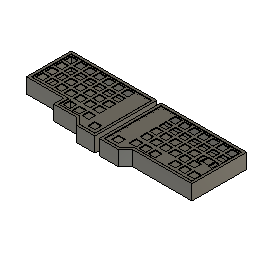
hwsplit (Autodesk Fusion 360 design; units mm, degrees)
Autodesk Fusion 360 part; units mm, degrees
sketch "Sketch1" plane through (0, 0, 0) normal (0, 0, 1) x (1, 0, 0)
  line L0 (3.025, -2.525) -> (16.025, -2.525)
  line L1 (3.025, -16.525) -> (16.025, -16.525)
  line L2 (2.525, -3.025) -> (2.525, -16.025)
  line L3 (16.525, -3.025) -> (16.525, -16.025)
  arc A0 (3.025, -2.525) -> (2.525, -3.025) centre (3.025, -3.025) ccw
  arc A1 (16.525, -3.025) -> (16.025, -2.525) centre (16.025, -3.025) ccw
  arc A2 (2.525, -16.025) -> (3.025, -16.525) centre (3.025, -16.025) ccw
  arc A3 (16.025, -16.525) -> (16.525, -16.025) centre (16.025, -16.025) ccw
  line L4 (22.075, -2.525) -> (35.075, -2.525)
  line L5 (22.075, -16.525) -> (35.075, -16.525)
  line L6 (21.575, -3.025) -> (21.575, -16.025)
  line L7 (35.575, -3.025) -> (35.575, -16.025)
  arc A4 (22.075, -2.525) -> (21.575, -3.025) centre (22.075, -3.025) ccw
  arc A5 (35.575, -3.025) -> (35.075, -2.525) centre (35.075, -3.025) ccw
  arc A6 (21.575, -16.025) -> (22.075, -16.525) centre (22.075, -16.025) ccw
  arc A7 (35.075, -16.525) -> (35.575, -16.025) centre (35.075, -16.025) ccw
  line L8 (41.125, -2.525) -> (54.125, -2.525)
  line L9 (41.125, -16.525) -> (54.125, -16.525)
  line L10 (40.625, -3.025) -> (40.625, -16.025)
  line L11 (54.625, -3.025) -> (54.625, -16.025)
  arc A8 (41.125, -2.525) -> (40.625, -3.025) centre (41.125, -3.025) ccw
  arc A9 (54.625, -3.025) -> (54.125, -2.525) centre (54.125, -3.025) ccw
  arc A10 (40.625, -16.025) -> (41.125, -16.525) centre (41.125, -16.025) ccw
  arc A11 (54.125, -16.525) -> (54.625, -16.025) centre (54.125, -16.025) ccw
  line L12 (60.175, -2.525) -> (73.175, -2.525)
  line L13 (60.175, -16.525) -> (73.175, -16.525)
  line L14 (59.675, -3.025) -> (59.675, -16.025)
  line L15 (73.675, -3.025) -> (73.675, -16.025)
  arc A12 (60.175, -2.525) -> (59.675, -3.025) centre (60.175, -3.025) ccw
  arc A13 (73.675, -3.025) -> (73.175, -2.525) centre (73.175, -3.025) ccw
  arc A14 (59.675, -16.025) -> (60.175, -16.525) centre (60.175, -16.025) ccw
  arc A15 (73.175, -16.525) -> (73.675, -16.025) centre (73.175, -16.025) ccw
  line L16 (79.225, -2.525) -> (92.225, -2.525)
  line L17 (79.225, -16.525) -> (92.225, -16.525)
  line L18 (78.725, -3.025) -> (78.725, -16.025)
  line L19 (92.725, -3.025) -> (92.725, -16.025)
  arc A16 (79.225, -2.525) -> (78.725, -3.025) centre (79.225, -3.025) ccw
  arc A17 (92.725, -3.025) -> (92.225, -2.525) centre (92.225, -3.025) ccw
  arc A18 (78.725, -16.025) -> (79.225, -16.525) centre (79.225, -16.025) ccw
  arc A19 (92.225, -16.525) -> (92.725, -16.025) centre (92.225, -16.025) ccw
  line L20 (98.275, -2.525) -> (111.275, -2.525)
  line L21 (98.275, -16.525) -> (111.275, -16.525)
  line L22 (97.775, -3.025) -> (97.775, -16.025)
  line L23 (111.775, -3.025) -> (111.775, -16.025)
  arc A20 (98.275, -2.525) -> (97.775, -3.025) centre (98.275, -3.025) ccw
  arc A21 (111.775, -3.025) -> (111.275, -2.525) centre (111.275, -3.025) ccw
  arc A22 (97.775, -16.025) -> (98.275, -16.525) centre (98.275, -16.025) ccw
  arc A23 (111.275, -16.525) -> (111.775, -16.025) centre (111.275, -16.025) ccw
  line L24 (117.325, -2.525) -> (130.325, -2.525)
  line L25 (117.325, -16.525) -> (130.325, -16.525)
  line L26 (116.825, -3.025) -> (116.825, -16.025)
  line L27 (130.825, -3.025) -> (130.825, -16.025)
  arc A24 (117.325, -2.525) -> (116.825, -3.025) centre (117.325, -3.025) ccw
  arc A25 (130.825, -3.025) -> (130.325, -2.525) centre (130.325, -3.025) ccw
  arc A26 (116.825, -16.025) -> (117.325, -16.525) centre (117.325, -16.025) ccw
  arc A27 (130.325, -16.525) -> (130.825, -16.025) centre (130.325, -16.025) ccw
  line L28 (212.575, -2.525) -> (225.575, -2.525)
  line L29 (212.575, -16.525) -> (225.575, -16.525)
  line L30 (212.075, -3.025) -> (212.075, -16.025)
  line L31 (226.075, -3.025) -> (226.075, -16.025)
  arc A28 (212.575, -2.525) -> (212.075, -3.025) centre (212.575, -3.025) ccw
  arc A29 (226.075, -3.025) -> (225.575, -2.525) centre (225.575, -3.025) ccw
  arc A30 (212.075, -16.025) -> (212.575, -16.525) centre (212.575, -16.025) ccw
  arc A31 (225.575, -16.525) -> (226.075, -16.025) centre (225.575, -16.025) ccw
  line L32 (231.625, -2.525) -> (244.625, -2.525)
  line L33 (231.625, -16.525) -> (244.625, -16.525)
  line L34 (231.125, -3.025) -> (231.125, -16.025)
  line L35 (245.125, -3.025) -> (245.125, -16.025)
  arc A32 (231.625, -2.525) -> (231.125, -3.025) centre (231.625, -3.025) ccw
  arc A33 (245.125, -3.025) -> (244.625, -2.525) centre (244.625, -3.025) ccw
  arc A34 (231.125, -16.025) -> (231.625, -16.525) centre (231.625, -16.025) ccw
  arc A35 (244.625, -16.525) -> (245.125, -16.025) centre (244.625, -16.025) ccw
  line L36 (250.675, -2.525) -> (263.675, -2.525)
  line L37 (250.675, -16.525) -> (263.675, -16.525)
  line L38 (250.175, -3.025) -> (250.175, -16.025)
  line L39 (264.175, -3.025) -> (264.175, -16.025)
  arc A36 (250.675, -2.525) -> (250.175, -3.025) centre (250.675, -3.025) ccw
  arc A37 (264.175, -3.025) -> (263.675, -2.525) centre (263.675, -3.025) ccw
  arc A38 (250.175, -16.025) -> (250.675, -16.525) centre (250.675, -16.025) ccw
  arc A39 (263.675, -16.525) -> (264.175, -16.025) centre (263.675, -16.025) ccw
  line L40 (269.725, -2.525) -> (282.725, -2.525)
  line L41 (269.725, -16.525) -> (282.725, -16.525)
  line L42 (269.225, -3.025) -> (269.225, -16.025)
  line L43 (283.225, -3.025) -> (283.225, -16.025)
  arc A40 (269.725, -2.525) -> (269.225, -3.025) centre (269.725, -3.025) ccw
  arc A41 (283.225, -3.025) -> (282.725, -2.525) centre (282.725, -3.025) ccw
  arc A42 (269.225, -16.025) -> (269.725, -16.525) centre (269.725, -16.025) ccw
  arc A43 (282.725, -16.525) -> (283.225, -16.025) centre (282.725, -16.025) ccw
  line L44 (288.775, -2.525) -> (301.775, -2.525)
  line L45 (288.775, -16.525) -> (301.775, -16.525)
  line L46 (288.275, -3.025) -> (288.275, -16.025)
  line L47 (302.275, -3.025) -> (302.275, -16.025)
  arc A44 (288.775, -2.525) -> (288.275, -3.025) centre (288.775, -3.025) ccw
  arc A45 (302.275, -3.025) -> (301.775, -2.525) centre (301.775, -3.025) ccw
  arc A46 (288.275, -16.025) -> (288.775, -16.525) centre (288.775, -16.025) ccw
  arc A47 (301.775, -16.525) -> (302.275, -16.025) centre (301.775, -16.025) ccw
  line L48 (307.825, -2.525) -> (320.825, -2.525)
  line L49 (307.825, -16.525) -> (320.825, -16.525)
  line L50 (307.325, -3.025) -> (307.325, -16.025)
  line L51 (321.325, -3.025) -> (321.325, -16.025)
  arc A48 (307.825, -2.525) -> (307.325, -3.025) centre (307.825, -3.025) ccw
  arc A49 (321.325, -3.025) -> (320.825, -2.525) centre (320.825, -3.025) ccw
  arc A50 (307.325, -16.025) -> (307.825, -16.525) centre (307.825, -16.025) ccw
  arc A51 (320.825, -16.525) -> (321.325, -16.025) centre (320.825, -16.025) ccw
  line L52 (326.875, -2.525) -> (339.875, -2.525)
  line L53 (326.875, -16.525) -> (339.875, -16.525)
  line L54 (326.375, -3.025) -> (326.375, -16.025)
  line L55 (340.375, -3.025) -> (340.375, -16.025)
  arc A52 (326.875, -2.525) -> (326.375, -3.025) centre (326.875, -3.025) ccw
  arc A53 (340.375, -3.025) -> (339.875, -2.525) centre (339.875, -3.025) ccw
  arc A54 (326.375, -16.025) -> (326.875, -16.525) centre (326.875, -16.025) ccw
  arc A55 (339.875, -16.525) -> (340.375, -16.025) centre (339.875, -16.025) ccw
  line L56 (3.025, -21.575) -> (16.025, -21.575)
  line L57 (3.025, -35.575) -> (16.025, -35.575)
  line L58 (2.525, -22.075) -> (2.525, -35.075)
  line L59 (16.525, -22.075) -> (16.525, -35.075)
  arc A56 (3.025, -21.575) -> (2.525, -22.075) centre (3.025, -22.075) ccw
  arc A57 (16.525, -22.075) -> (16.025, -21.575) centre (16.025, -22.075) ccw
  arc A58 (2.525, -35.075) -> (3.025, -35.575) centre (3.025, -35.075) ccw
  arc A59 (16.025, -35.575) -> (16.525, -35.075) centre (16.025, -35.075) ccw
  line L60 (22.075, -21.575) -> (35.075, -21.575)
  line L61 (22.075, -35.575) -> (35.075, -35.575)
  line L62 (21.575, -22.075) -> (21.575, -35.075)
  line L63 (35.575, -22.075) -> (35.575, -35.075)
  arc A60 (22.075, -21.575) -> (21.575, -22.075) centre (22.075, -22.075) ccw
  arc A61 (35.575, -22.075) -> (35.075, -21.575) centre (35.075, -22.075) ccw
  arc A62 (21.575, -35.075) -> (22.075, -35.575) centre (22.075, -35.075) ccw
  arc A63 (35.075, -35.575) -> (35.575, -35.075) centre (35.075, -35.075) ccw
  line L64 (41.125, -21.575) -> (54.125, -21.575)
  line L65 (41.125, -35.575) -> (54.125, -35.575)
  line L66 (40.625, -22.075) -> (40.625, -35.075)
  line L67 (54.625, -22.075) -> (54.625, -35.075)
  arc A64 (41.125, -21.575) -> (40.625, -22.075) centre (41.125, -22.075) ccw
  arc A65 (54.625, -22.075) -> (54.125, -21.575) centre (54.125, -22.075) ccw
  arc A66 (40.625, -35.075) -> (41.125, -35.575) centre (41.125, -35.075) ccw
  arc A67 (54.125, -35.575) -> (54.625, -35.075) centre (54.125, -35.075) ccw
  line L68 (60.175, -21.575) -> (73.175, -21.575)
  line L69 (60.175, -35.575) -> (73.175, -35.575)
  line L70 (59.675, -22.075) -> (59.675, -35.075)
  line L71 (73.675, -22.075) -> (73.675, -35.075)
  arc A68 (60.175, -21.575) -> (59.675, -22.075) centre (60.175, -22.075) ccw
  arc A69 (73.675, -22.075) -> (73.175, -21.575) centre (73.175, -22.075) ccw
  arc A70 (59.675, -35.075) -> (60.175, -35.575) centre (60.175, -35.075) ccw
  arc A71 (73.175, -35.575) -> (73.675, -35.075) centre (73.175, -35.075) ccw
  line L72 (79.225, -21.575) -> (92.225, -21.575)
  line L73 (79.225, -35.575) -> (92.225, -35.575)
  line L74 (78.725, -22.075) -> (78.725, -35.075)
  line L75 (92.725, -22.075) -> (92.725, -35.075)
  arc A72 (79.225, -21.575) -> (78.725, -22.075) centre (79.225, -22.075) ccw
  arc A73 (92.725, -22.075) -> (92.225, -21.575) centre (92.225, -22.075) ccw
  arc A74 (78.725, -35.075) -> (79.225, -35.575) centre (79.225, -35.075) ccw
  arc A75 (92.225, -35.575) -> (92.725, -35.075) centre (92.225, -35.075) ccw
  line L76 (98.275, -21.575) -> (111.275, -21.575)
  line L77 (98.275, -35.575) -> (111.275, -35.575)
  line L78 (97.775, -22.075) -> (97.775, -35.075)
  line L79 (111.775, -22.075) -> (111.775, -35.075)
  arc A76 (98.275, -21.575) -> (97.775, -22.075) centre (98.275, -22.075) ccw
  arc A77 (111.775, -22.075) -> (111.275, -21.575) centre (111.275, -22.075) ccw
  arc A78 (97.775, -35.075) -> (98.275, -35.575) centre (98.275, -35.075) ccw
  arc A79 (111.275, -35.575) -> (111.775, -35.075) centre (111.275, -35.075) ccw
  line L80 (117.325, -21.575) -> (130.325, -21.575)
  line L81 (117.325, -35.575) -> (130.325, -35.575)
  line L82 (116.825, -22.075) -> (116.825, -35.075)
  line L83 (130.825, -22.075) -> (130.825, -35.075)
  arc A80 (117.325, -21.575) -> (116.825, -22.075) centre (117.325, -22.075) ccw
  arc A81 (130.825, -22.075) -> (130.325, -21.575) centre (130.325, -22.075) ccw
  arc A82 (116.825, -35.075) -> (117.325, -35.575) centre (117.325, -35.075) ccw
  arc A83 (130.325, -35.575) -> (130.825, -35.075) centre (130.325, -35.075) ccw
  line L84 (212.575, -21.575) -> (225.575, -21.575)
  line L85 (212.575, -35.575) -> (225.575, -35.575)
  line L86 (212.075, -22.075) -> (212.075, -35.075)
  line L87 (226.075, -22.075) -> (226.075, -35.075)
  arc A84 (212.575, -21.575) -> (212.075, -22.075) centre (212.575, -22.075) ccw
  arc A85 (226.075, -22.075) -> (225.575, -21.575) centre (225.575, -22.075) ccw
  arc A86 (212.075, -35.075) -> (212.575, -35.575) centre (212.575, -35.075) ccw
  arc A87 (225.575, -35.575) -> (226.075, -35.075) centre (225.575, -35.075) ccw
  line L88 (231.625, -21.575) -> (244.625, -21.575)
  line L89 (231.625, -35.575) -> (244.625, -35.575)
  line L90 (231.125, -22.075) -> (231.125, -35.075)
  line L91 (245.125, -22.075) -> (245.125, -35.075)
  arc A88 (231.625, -21.575) -> (231.125, -22.075) centre (231.625, -22.075) ccw
  arc A89 (245.125, -22.075) -> (244.625, -21.575) centre (244.625, -22.075) ccw
  arc A90 (231.125, -35.075) -> (231.625, -35.575) centre (231.625, -35.075) ccw
  arc A91 (244.625, -35.575) -> (245.125, -35.075) centre (244.625, -35.075) ccw
  line L92 (250.675, -21.575) -> (263.675, -21.575)
  line L93 (250.675, -35.575) -> (263.675, -35.575)
  line L94 (250.175, -22.075) -> (250.175, -35.075)
  line L95 (264.175, -22.075) -> (264.175, -35.075)
  arc A92 (250.675, -21.575) -> (250.175, -22.075) centre (250.675, -22.075) ccw
  arc A93 (264.175, -22.075) -> (263.675, -21.575) centre (263.675, -22.075) ccw
  arc A94 (250.175, -35.075) -> (250.675, -35.575) centre (250.675, -35.075) ccw
  arc A95 (263.675, -35.575) -> (264.175, -35.075) centre (263.675, -35.075) ccw
  line L96 (269.725, -21.575) -> (282.725, -21.575)
  line L97 (269.725, -35.575) -> (282.725, -35.575)
  line L98 (269.225, -22.075) -> (269.225, -35.075)
  line L99 (283.225, -22.075) -> (283.225, -35.075)
  arc A96 (269.725, -21.575) -> (269.225, -22.075) centre (269.725, -22.075) ccw
  arc A97 (283.225, -22.075) -> (282.725, -21.575) centre (282.725, -22.075) ccw
  arc A98 (269.225, -35.075) -> (269.725, -35.575) centre (269.725, -35.075) ccw
  arc A99 (282.725, -35.575) -> (283.225, -35.075) centre (282.725, -35.075) ccw
  line L100 (288.775, -21.575) -> (301.775, -21.575)
  line L101 (288.775, -35.575) -> (301.775, -35.575)
  line L102 (288.275, -22.075) -> (288.275, -35.075)
  line L103 (302.275, -22.075) -> (302.275, -35.075)
  arc A100 (288.775, -21.575) -> (288.275, -22.075) centre (288.775, -22.075) ccw
  arc A101 (302.275, -22.075) -> (301.775, -21.575) centre (301.775, -22.075) ccw
  arc A102 (288.275, -35.075) -> (288.775, -35.575) centre (288.775, -35.075) ccw
  arc A103 (301.775, -35.575) -> (302.275, -35.075) centre (301.775, -35.075) ccw
  line L104 (307.825, -21.575) -> (320.825, -21.575)
  line L105 (307.825, -35.575) -> (320.825, -35.575)
  line L106 (307.325, -22.075) -> (307.325, -35.075)
  line L107 (321.325, -22.075) -> (321.325, -35.075)
  arc A104 (307.825, -21.575) -> (307.325, -22.075) centre (307.825, -22.075) ccw
  arc A105 (321.325, -22.075) -> (320.825, -21.575) centre (320.825, -22.075) ccw
  arc A106 (307.325, -35.075) -> (307.825, -35.575) centre (307.825, -35.075) ccw
  arc A107 (320.825, -35.575) -> (321.325, -35.075) centre (320.825, -35.075) ccw
  line L108 (326.875, -21.575) -> (339.875, -21.575)
  line L109 (326.875, -35.575) -> (339.875, -35.575)
  line L110 (326.375, -22.075) -> (326.375, -35.075)
  line L111 (340.375, -22.075) -> (340.375, -35.075)
  arc A108 (326.875, -21.575) -> (326.375, -22.075) centre (326.875, -22.075) ccw
  arc A109 (340.375, -22.075) -> (339.875, -21.575) centre (339.875, -22.075) ccw
  arc A110 (326.375, -35.075) -> (326.875, -35.575) centre (326.875, -35.075) ccw
  arc A111 (339.875, -35.575) -> (340.375, -35.075) centre (339.875, -35.075) ccw
  line L112 (3.025, -40.625) -> (16.025, -40.625)
  line L113 (3.025, -54.625) -> (16.025, -54.625)
  line L114 (2.525, -41.125) -> (2.525, -54.125)
  line L115 (16.525, -41.125) -> (16.525, -54.125)
  arc A112 (3.025, -40.625) -> (2.525, -41.125) centre (3.025, -41.125) ccw
  arc A113 (16.525, -41.125) -> (16.025, -40.625) centre (16.025, -41.125) ccw
  arc A114 (2.525, -54.125) -> (3.025, -54.625) centre (3.025, -54.125) ccw
  arc A115 (16.025, -54.625) -> (16.525, -54.125) centre (16.025, -54.125) ccw
  line L116 (22.075, -40.625) -> (35.075, -40.625)
  line L117 (22.075, -54.625) -> (35.075, -54.625)
  line L118 (21.575, -41.125) -> (21.575, -54.125)
  line L119 (35.575, -41.125) -> (35.575, -54.125)
  arc A116 (22.075, -40.625) -> (21.575, -41.125) centre (22.075, -41.125) ccw
  arc A117 (35.575, -41.125) -> (35.075, -40.625) centre (35.075, -41.125) ccw
  arc A118 (21.575, -54.125) -> (22.075, -54.625) centre (22.075, -54.125) ccw
  arc A119 (35.075, -54.625) -> (35.575, -54.125) centre (35.075, -54.125) ccw
  line L120 (41.125, -40.625) -> (54.125, -40.625)
  line L121 (41.125, -54.625) -> (54.125, -54.625)
  line L122 (40.625, -41.125) -> (40.625, -54.125)
  line L123 (54.625, -41.125) -> (54.625, -54.125)
  arc A120 (41.125, -40.625) -> (40.625, -41.125) centre (41.125, -41.125) ccw
  arc A121 (54.625, -41.125) -> (54.125, -40.625) centre (54.125, -41.125) ccw
  arc A122 (40.625, -54.125) -> (41.125, -54.625) centre (41.125, -54.125) ccw
  arc A123 (54.125, -54.625) -> (54.625, -54.125) centre (54.125, -54.125) ccw
  line L124 (60.175, -40.625) -> (73.175, -40.625)
  line L125 (60.175, -54.625) -> (73.175, -54.625)
  line L126 (59.675, -41.125) -> (59.675, -54.125)
  line L127 (73.675, -41.125) -> (73.675, -54.125)
  arc A124 (60.175, -40.625) -> (59.675, -41.125) centre (60.175, -41.125) ccw
  arc A125 (73.675, -41.125) -> (73.175, -40.625) centre (73.175, -41.125) ccw
  arc A126 (59.675, -54.125) -> (60.175, -54.625) centre (60.175, -54.125) ccw
  arc A127 (73.175, -54.625) -> (73.675, -54.125) centre (73.175, -54.125) ccw
  line L128 (79.225, -40.625) -> (92.225, -40.625)
  line L129 (79.225, -54.625) -> (92.225, -54.625)
  line L130 (78.725, -41.125) -> (78.725, -54.125)
  line L131 (92.725, -41.125) -> (92.725, -54.125)
  arc A128 (79.225, -40.625) -> (78.725, -41.125) centre (79.225, -41.125) ccw
  arc A129 (92.725, -41.125) -> (92.225, -40.625) centre (92.225, -41.125) ccw
  arc A130 (78.725, -54.125) -> (79.225, -54.625) centre (79.225, -54.125) ccw
  arc A131 (92.225, -54.625) -> (92.725, -54.125) centre (92.225, -54.125) ccw
  line L132 (98.275, -40.625) -> (111.275, -40.625)
  line L133 (98.275, -54.625) -> (111.275, -54.625)
  line L134 (97.775, -41.125) -> (97.775, -54.125)
  line L135 (111.775, -41.125) -> (111.775, -54.125)
  arc A132 (98.275, -40.625) -> (97.775, -41.125) centre (98.275, -41.125) ccw
  arc A133 (111.775, -41.125) -> (111.275, -40.625) centre (111.275, -41.125) ccw
  arc A134 (97.775, -54.125) -> (98.275, -54.625) centre (98.275, -54.125) ccw
  arc A135 (111.275, -54.625) -> (111.775, -54.125) centre (111.275, -54.125) ccw
  line L136 (117.325, -40.625) -> (130.325, -40.625)
  line L137 (117.325, -54.625) -> (130.325, -54.625)
  line L138 (116.825, -41.125) -> (116.825, -54.125)
  line L139 (130.825, -41.125) -> (130.825, -54.125)
  arc A136 (117.325, -40.625) -> (116.825, -41.125) centre (117.325, -41.125) ccw
  arc A137 (130.825, -41.125) -> (130.325, -40.625) centre (130.325, -41.125) ccw
  arc A138 (116.825, -54.125) -> (117.325, -54.625) centre (117.325, -54.125) ccw
  arc A139 (130.325, -54.625) -> (130.825, -54.125) centre (130.325, -54.125) ccw
  line L140 (212.575, -40.625) -> (225.575, -40.625)
  line L141 (212.575, -54.625) -> (225.575, -54.625)
  line L142 (212.075, -41.125) -> (212.075, -54.125)
  line L143 (226.075, -41.125) -> (226.075, -54.125)
  arc A140 (212.575, -40.625) -> (212.075, -41.125) centre (212.575, -41.125) ccw
  arc A141 (226.075, -41.125) -> (225.575, -40.625) centre (225.575, -41.125) ccw
  arc A142 (212.075, -54.125) -> (212.575, -54.625) centre (212.575, -54.125) ccw
  arc A143 (225.575, -54.625) -> (226.075, -54.125) centre (225.575, -54.125) ccw
  line L144 (231.625, -40.625) -> (244.625, -40.625)
  line L145 (231.625, -54.625) -> (244.625, -54.625)
  line L146 (231.125, -41.125) -> (231.125, -54.125)
  line L147 (245.125, -41.125) -> (245.125, -54.125)
  arc A144 (231.625, -40.625) -> (231.125, -41.125) centre (231.625, -41.125) ccw
  arc A145 (245.125, -41.125) -> (244.625, -40.625) centre (244.625, -41.125) ccw
  arc A146 (231.125, -54.125) -> (231.625, -54.625) centre (231.625, -54.125) ccw
  arc A147 (244.625, -54.625) -> (245.125, -54.125) centre (244.625, -54.125) ccw
  line L148 (250.675, -40.625) -> (263.675, -40.625)
  line L149 (250.675, -54.625) -> (263.675, -54.625)
  line L150 (250.175, -41.125) -> (250.175, -54.125)
  line L151 (264.175, -41.125) -> (264.175, -54.125)
  arc A148 (250.675, -40.625) -> (250.175, -41.125) centre (250.675, -41.125) ccw
  arc A149 (264.175, -41.125) -> (263.675, -40.625) centre (263.675, -41.125) ccw
  arc A150 (250.175, -54.125) -> (250.675, -54.625) centre (250.675, -54.125) ccw
  arc A151 (263.675, -54.625) -> (264.175, -54.125) centre (263.675, -54.125) ccw
  line L152 (269.725, -40.625) -> (282.725, -40.625)
  line L153 (269.725, -54.625) -> (282.725, -54.625)
  line L154 (269.225, -41.125) -> (269.225, -54.125)
  line L155 (283.225, -41.125) -> (283.225, -54.125)
  arc A152 (269.725, -40.625) -> (269.225, -41.125) centre (269.725, -41.125) ccw
  arc A153 (283.225, -41.125) -> (282.725, -40.625) centre (282.725, -41.125) ccw
  arc A154 (269.225, -54.125) -> (269.725, -54.625) centre (269.725, -54.125) ccw
  arc A155 (282.725, -54.625) -> (283.225, -54.125) centre (282.725, -54.125) ccw
  line L156 (288.775, -40.625) -> (301.775, -40.625)
  line L157 (288.775, -54.625) -> (301.775, -54.625)
  line L158 (288.275, -41.125) -> (288.275, -54.125)
  line L159 (302.275, -41.125) -> (302.275, -54.125)
  arc A156 (288.775, -40.625) -> (288.275, -41.125) centre (288.775, -41.125) ccw
  arc A157 (302.275, -41.125) -> (301.775, -40.625) centre (301.775, -41.125) ccw
  arc A158 (288.275, -54.125) -> (288.775, -54.625) centre (288.775, -54.125) ccw
  arc A159 (301.775, -54.625) -> (302.275, -54.125) centre (301.775, -54.125) ccw
  line L160 (317.35, -40.625) -> (330.35, -40.625)
  line L161 (317.35, -54.625) -> (330.35, -54.625)
  line L162 (316.85, -41.125) -> (316.85, -54.125)
  line L163 (330.85, -41.125) -> (330.85, -54.125)
  arc A160 (317.35, -40.625) -> (316.85, -41.125) centre (317.35, -41.125) ccw
  arc A161 (330.85, -41.125) -> (330.35, -40.625) centre (330.35, -41.125) ccw
  arc A162 (316.85, -54.125) -> (317.35, -54.625) centre (317.35, -54.125) ccw
  arc A163 (330.35, -54.625) -> (330.85, -54.125) centre (330.35, -54.125) ccw
  line L164 (308.912, -41.625) -> (314.912, -41.625)
  line L165 (308.912, -56.625) -> (314.912, -56.625)
  line L166 (308.412, -42.125) -> (308.412, -56.125)
  line L167 (315.412, -42.125) -> (315.412, -56.125)
  arc A164 (308.912, -41.625) -> (308.412, -42.125) centre (308.912, -42.125) ccw
  arc A165 (315.412, -42.125) -> (314.912, -41.625) centre (314.912, -42.125) ccw
  arc A166 (308.412, -56.125) -> (308.912, -56.625) centre (308.912, -56.125) ccw
  arc A167 (314.912, -56.625) -> (315.412, -56.125) centre (314.912, -56.125) ccw
  line L168 (332.788, -41.625) -> (338.788, -41.625)
  line L169 (332.788, -56.625) -> (338.788, -56.625)
  line L170 (332.288, -42.125) -> (332.288, -56.125)
  line L171 (339.288, -42.125) -> (339.288, -56.125)
  arc A168 (332.788, -41.625) -> (332.288, -42.125) centre (332.788, -42.125) ccw
  arc A169 (339.288, -42.125) -> (338.788, -41.625) centre (338.788, -42.125) ccw
  arc A170 (332.288, -56.125) -> (332.788, -56.625) centre (332.788, -56.125) ccw
  arc A171 (338.788, -56.625) -> (339.288, -56.125) centre (338.788, -56.125) ccw
  line L172 (3.025, -59.675) -> (16.025, -59.675)
  line L173 (3.025, -73.675) -> (16.025, -73.675)
  line L174 (2.525, -60.175) -> (2.525, -73.175)
  line L175 (16.525, -60.175) -> (16.525, -73.175)
  arc A172 (3.025, -59.675) -> (2.525, -60.175) centre (3.025, -60.175) ccw
  arc A173 (16.525, -60.175) -> (16.025, -59.675) centre (16.025, -60.175) ccw
  arc A174 (2.525, -73.175) -> (3.025, -73.675) centre (3.025, -73.175) ccw
  arc A175 (16.025, -73.675) -> (16.525, -73.175) centre (16.025, -73.175) ccw
  line L176 (22.075, -59.675) -> (35.075, -59.675)
  line L177 (22.075, -73.675) -> (35.075, -73.675)
  line L178 (21.575, -60.175) -> (21.575, -73.175)
  line L179 (35.575, -60.175) -> (35.575, -73.175)
  arc A176 (22.075, -59.675) -> (21.575, -60.175) centre (22.075, -60.175) ccw
  arc A177 (35.575, -60.175) -> (35.075, -59.675) centre (35.075, -60.175) ccw
  arc A178 (21.575, -73.175) -> (22.075, -73.675) centre (22.075, -73.175) ccw
  arc A179 (35.075, -73.675) -> (35.575, -73.175) centre (35.075, -73.175) ccw
  line L180 (41.125, -59.675) -> (54.125, -59.675)
  line L181 (41.125, -73.675) -> (54.125, -73.675)
  line L182 (40.625, -60.175) -> (40.625, -73.175)
  line L183 (54.625, -60.175) -> (54.625, -73.175)
  arc A180 (41.125, -59.675) -> (40.625, -60.175) centre (41.125, -60.175) ccw
  arc A181 (54.625, -60.175) -> (54.125, -59.675) centre (54.125, -60.175) ccw
  arc A182 (40.625, -73.175) -> (41.125, -73.675) centre (41.125, -73.175) ccw
  arc A183 (54.125, -73.675) -> (54.625, -73.175) centre (54.125, -73.175) ccw
  line L184 (60.175, -59.675) -> (73.175, -59.675)
  line L185 (60.175, -73.675) -> (73.175, -73.675)
  line L186 (59.675, -60.175) -> (59.675, -73.175)
  line L187 (73.675, -60.175) -> (73.675, -73.175)
  arc A184 (60.175, -59.675) -> (59.675, -60.175) centre (60.175, -60.175) ccw
  arc A185 (73.675, -60.175) -> (73.175, -59.675) centre (73.175, -60.175) ccw
  arc A186 (59.675, -73.175) -> (60.175, -73.675) centre (60.175, -73.175) ccw
  arc A187 (73.175, -73.675) -> (73.675, -73.175) centre (73.175, -73.175) ccw
  line L188 (79.225, -59.675) -> (92.225, -59.675)
  line L189 (79.225, -73.675) -> (92.225, -73.675)
  line L190 (78.725, -60.175) -> (78.725, -73.175)
  line L191 (92.725, -60.175) -> (92.725, -73.175)
  arc A188 (79.225, -59.675) -> (78.725, -60.175) centre (79.225, -60.175) ccw
  arc A189 (92.725, -60.175) -> (92.225, -59.675) centre (92.225, -60.175) ccw
  arc A190 (78.725, -73.175) -> (79.225, -73.675) centre (79.225, -73.175) ccw
  arc A191 (92.225, -73.675) -> (92.725, -73.175) centre (92.225, -73.175) ccw
  line L192 (98.275, -59.675) -> (111.275, -59.675)
  line L193 (98.275, -73.675) -> (111.275, -73.675)
  line L194 (97.775, -60.175) -> (97.775, -73.175)
  line L195 (111.775, -60.175) -> (111.775, -73.175)
  arc A192 (98.275, -59.675) -> (97.775, -60.175) centre (98.275, -60.175) ccw
  arc A193 (111.775, -60.175) -> (111.275, -59.675) centre (111.275, -60.175) ccw
  arc A194 (97.775, -73.175) -> (98.275, -73.675) centre (98.275, -73.175) ccw
  arc A195 (111.275, -73.675) -> (111.775, -73.175) centre (111.275, -73.175) ccw
  line L196 (117.325, -59.675) -> (130.325, -59.675)
  line L197 (117.325, -73.675) -> (130.325, -73.675)
  line L198 (116.825, -60.175) -> (116.825, -73.175)
  line L199 (130.825, -60.175) -> (130.825, -73.175)
  arc A196 (117.325, -59.675) -> (116.825, -60.175) centre (117.325, -60.175) ccw
  arc A197 (130.825, -60.175) -> (130.325, -59.675) centre (130.325, -60.175) ccw
  arc A198 (116.825, -73.175) -> (117.325, -73.675) centre (117.325, -73.175) ccw
  arc A199 (130.325, -73.675) -> (130.825, -73.175) centre (130.325, -73.175) ccw
  line L200 (212.575, -59.675) -> (225.575, -59.675)
  line L201 (212.575, -73.675) -> (225.575, -73.675)
  line L202 (212.075, -60.175) -> (212.075, -73.175)
  line L203 (226.075, -60.175) -> (226.075, -73.175)
  arc A200 (212.575, -59.675) -> (212.075, -60.175) centre (212.575, -60.175) ccw
  arc A201 (226.075, -60.175) -> (225.575, -59.675) centre (225.575, -60.175) ccw
  arc A202 (212.075, -73.175) -> (212.575, -73.675) centre (212.575, -73.175) ccw
  arc A203 (225.575, -73.675) -> (226.075, -73.175) centre (225.575, -73.175) ccw
  line L204 (231.625, -59.675) -> (244.625, -59.675)
  line L205 (231.625, -73.675) -> (244.625, -73.675)
  line L206 (231.125, -60.175) -> (231.125, -73.175)
  line L207 (245.125, -60.175) -> (245.125, -73.175)
  arc A204 (231.625, -59.675) -> (231.125, -60.175) centre (231.625, -60.175) ccw
  arc A205 (245.125, -60.175) -> (244.625, -59.675) centre (244.625, -60.175) ccw
  arc A206 (231.125, -73.175) -> (231.625, -73.675) centre (231.625, -73.175) ccw
  arc A207 (244.625, -73.675) -> (245.125, -73.175) centre (244.625, -73.175) ccw
  line L208 (250.675, -59.675) -> (263.675, -59.675)
  line L209 (250.675, -73.675) -> (263.675, -73.675)
  line L210 (250.175, -60.175) -> (250.175, -73.175)
  line L211 (264.175, -60.175) -> (264.175, -73.175)
  arc A208 (250.675, -59.675) -> (250.175, -60.175) centre (250.675, -60.175) ccw
  arc A209 (264.175, -60.175) -> (263.675, -59.675) centre (263.675, -60.175) ccw
  arc A210 (250.175, -73.175) -> (250.675, -73.675) centre (250.675, -73.175) ccw
  arc A211 (263.675, -73.675) -> (264.175, -73.175) centre (263.675, -73.175) ccw
  line L212 (269.725, -59.675) -> (282.725, -59.675)
  line L213 (269.725, -73.675) -> (282.725, -73.675)
  line L214 (269.225, -60.175) -> (269.225, -73.175)
  line L215 (283.225, -60.175) -> (283.225, -73.175)
  arc A212 (269.725, -59.675) -> (269.225, -60.175) centre (269.725, -60.175) ccw
  arc A213 (283.225, -60.175) -> (282.725, -59.675) centre (282.725, -60.175) ccw
  arc A214 (269.225, -73.175) -> (269.725, -73.675) centre (269.725, -73.175) ccw
  arc A215 (282.725, -73.675) -> (283.225, -73.175) centre (282.725, -73.175) ccw
  line L216 (288.775, -59.675) -> (301.775, -59.675)
  line L217 (288.775, -73.675) -> (301.775, -73.675)
  line L218 (288.275, -60.175) -> (288.275, -73.175)
  line L219 (302.275, -60.175) -> (302.275, -73.175)
  arc A216 (288.775, -59.675) -> (288.275, -60.175) centre (288.775, -60.175) ccw
  arc A217 (302.275, -60.175) -> (301.775, -59.675) centre (301.775, -60.175) ccw
  arc A218 (288.275, -73.175) -> (288.775, -73.675) centre (288.775, -73.175) ccw
  arc A219 (301.775, -73.675) -> (302.275, -73.175) centre (301.775, -73.175) ccw
  line L220 (307.825, -59.675) -> (320.825, -59.675)
  line L221 (307.825, -73.675) -> (320.825, -73.675)
  line L222 (307.325, -60.175) -> (307.325, -73.175)
  line L223 (321.325, -60.175) -> (321.325, -73.175)
  arc A220 (307.825, -59.675) -> (307.325, -60.175) centre (307.825, -60.175) ccw
  arc A221 (321.325, -60.175) -> (320.825, -59.675) centre (320.825, -60.175) ccw
  arc A222 (307.325, -73.175) -> (307.825, -73.675) centre (307.825, -73.175) ccw
  arc A223 (320.825, -73.675) -> (321.325, -73.175) centre (320.825, -73.175) ccw
  line L224 (92.725, -81.6063) -> (92.725, -94.6063)
  line L225 (78.725, -81.6063) -> (78.725, -94.6063)
  line L226 (92.225, -81.1063) -> (79.225, -81.1063)
  line L227 (92.225, -95.1063) -> (79.225, -95.1063)
  arc A224 (92.725, -81.6063) -> (92.225, -81.1063) centre (92.225, -81.6063) ccw
  arc A225 (92.225, -95.1063) -> (92.725, -94.6063) centre (92.225, -94.6063) ccw
  arc A226 (79.225, -81.1063) -> (78.725, -81.6063) centre (79.225, -81.6063) ccw
  arc A227 (78.725, -94.6063) -> (79.225, -95.1063) centre (79.225, -94.6063) ccw
  line L228 (111.775, -81.6063) -> (111.775, -94.6063)
  line L229 (97.775, -81.6063) -> (97.775, -94.6063)
  line L230 (111.275, -81.1063) -> (98.275, -81.1063)
  line L231 (111.275, -95.1063) -> (98.275, -95.1063)
  arc A228 (111.775, -81.6063) -> (111.275, -81.1063) centre (111.275, -81.6063) ccw
  arc A229 (111.275, -95.1063) -> (111.775, -94.6063) centre (111.275, -94.6063) ccw
  arc A230 (98.275, -81.1063) -> (97.775, -81.6063) centre (98.275, -81.6063) ccw
  arc A231 (97.775, -94.6063) -> (98.275, -95.1062) centre (98.275, -94.6063) ccw
  line L232 (130.825, -81.6063) -> (130.825, -94.6063)
  line L233 (116.825, -81.6063) -> (116.825, -94.6063)
  line L234 (130.325, -81.1063) -> (117.325, -81.1063)
  line L235 (130.325, -95.1063) -> (117.325, -95.1063)
  arc A232 (130.825, -81.6063) -> (130.325, -81.1063) centre (130.325, -81.6063) ccw
  arc A233 (130.325, -95.1063) -> (130.825, -94.6063) centre (130.325, -94.6063) ccw
  arc A234 (117.325, -81.1063) -> (116.825, -81.6063) centre (117.325, -81.6063) ccw
  arc A235 (116.825, -94.6063) -> (117.325, -95.1063) centre (117.325, -94.6063) ccw
  line L236 (226.075, -81.6063) -> (226.075, -94.6063)
  line L237 (212.075, -81.6063) -> (212.075, -94.6063)
  line L238 (225.575, -81.1063) -> (212.575, -81.1063)
  line L239 (225.575, -95.1063) -> (212.575, -95.1063)
  arc A236 (226.075, -81.6063) -> (225.575, -81.1063) centre (225.575, -81.6063) ccw
  arc A237 (225.575, -95.1063) -> (226.075, -94.6063) centre (225.575, -94.6063) ccw
  arc A238 (212.575, -81.1063) -> (212.075, -81.6063) centre (212.575, -81.6063) ccw
  arc A239 (212.075, -94.6063) -> (212.575, -95.1063) centre (212.575, -94.6063) ccw
  line L240 (245.125, -81.6063) -> (245.125, -94.6063)
  line L241 (231.125, -81.6063) -> (231.125, -94.6063)
  line L242 (244.625, -81.1063) -> (231.625, -81.1063)
  line L243 (244.625, -95.1063) -> (231.625, -95.1063)
  arc A240 (245.125, -81.6063) -> (244.625, -81.1063) centre (244.625, -81.6063) ccw
  arc A241 (244.625, -95.1063) -> (245.125, -94.6063) centre (244.625, -94.6063) ccw
  arc A242 (231.625, -81.1063) -> (231.125, -81.6063) centre (231.625, -81.6063) ccw
  arc A243 (231.125, -94.6063) -> (231.625, -95.1063) centre (231.625, -94.6063) ccw
  line L244 (264.175, -81.6063) -> (264.175, -94.6063)
  line L245 (250.175, -81.6063) -> (250.175, -94.6063)
  line L246 (263.675, -81.1063) -> (250.675, -81.1063)
  line L247 (263.675, -95.1063) -> (250.675, -95.1063)
  arc A244 (264.175, -81.6063) -> (263.675, -81.1063) centre (263.675, -81.6063) ccw
  arc A245 (263.675, -95.1063) -> (264.175, -94.6063) centre (263.675, -94.6063) ccw
  arc A246 (250.675, -81.1063) -> (250.175, -81.6063) centre (250.675, -81.6063) ccw
  arc A247 (250.175, -94.6063) -> (250.675, -95.1063) centre (250.675, -94.6063) ccw
  line L248 (288.775, -78.725) -> (301.775, -78.725)
  line L249 (288.775, -92.725) -> (301.775, -92.725)
  line L250 (288.275, -79.225) -> (288.275, -92.225)
  line L251 (302.275, -79.225) -> (302.275, -92.225)
  arc A248 (288.775, -78.725) -> (288.275, -79.225) centre (288.775, -79.225) ccw
  arc A249 (302.275, -79.225) -> (301.775, -78.725) centre (301.775, -79.225) ccw
  arc A250 (288.275, -92.225) -> (288.775, -92.725) centre (288.775, -92.225) ccw
  arc A251 (301.775, -92.725) -> (302.275, -92.225) centre (301.775, -92.225) ccw
  line L252 (307.825, -78.725) -> (320.825, -78.725)
  line L253 (307.825, -92.725) -> (320.825, -92.725)
  line L254 (307.325, -79.225) -> (307.325, -92.225)
  line L255 (321.325, -79.225) -> (321.325, -92.225)
  arc A252 (307.825, -78.725) -> (307.325, -79.225) centre (307.825, -79.225) ccw
  arc A253 (321.325, -79.225) -> (320.825, -78.725) centre (320.825, -79.225) ccw
  arc A254 (307.325, -92.225) -> (307.825, -92.725) centre (307.825, -92.225) ccw
  arc A255 (320.825, -92.725) -> (321.325, -92.225) centre (320.825, -92.225) ccw
  line L256 (326.875, -78.725) -> (339.875, -78.725)
  line L257 (326.875, -92.725) -> (339.875, -92.725)
  line L258 (326.375, -79.225) -> (326.375, -92.225)
  line L259 (340.375, -79.225) -> (340.375, -92.225)
  arc A256 (326.875, -78.725) -> (326.375, -79.225) centre (326.875, -79.225) ccw
  arc A257 (340.375, -79.225) -> (339.875, -78.725) centre (339.875, -79.225) ccw
  arc A258 (326.375, -92.225) -> (326.875, -92.725) centre (326.875, -92.225) ccw
  arc A259 (339.875, -92.725) -> (340.375, -92.225) centre (339.875, -92.225) ccw
  line L260 (141.1375, -93.0125) -> (154.1375, -93.0125)
  line L261 (141.1375, -107.0125) -> (154.1375, -107.0125)
  line L262 (140.6375, -93.5125) -> (140.6375, -106.5125)
  line L263 (154.6375, -93.5125) -> (154.6375, -106.5125)
  arc A260 (141.1375, -93.0125) -> (140.6375, -93.5125) centre (141.1375, -93.5125) ccw
  arc A261 (154.6375, -93.5125) -> (154.1375, -93.0125) centre (154.1375, -93.5125) ccw
  arc A262 (140.6375, -106.5125) -> (141.1375, -107.0125) centre (141.1375, -106.5125) ccw
  arc A263 (154.1375, -107.0125) -> (154.6375, -106.5125) centre (154.1375, -106.5125) ccw
  line L264 (188.7625, -93.0125) -> (201.7625, -93.0125)
  line L265 (188.7625, -107.0125) -> (201.7625, -107.0125)
  line L266 (188.2625, -93.5125) -> (188.2625, -106.5125)
  line L267 (202.2625, -93.5125) -> (202.2625, -106.5125)
  arc A264 (188.7625, -93.0125) -> (188.2625, -93.5125) centre (188.7625, -93.5125) ccw
  arc A265 (202.2625, -93.5125) -> (201.7625, -93.0125) centre (201.7625, -93.5125) ccw
  arc A266 (188.2625, -106.5125) -> (188.7625, -107.0125) centre (188.7625, -106.5125) ccw
  arc A267 (201.7625, -107.0125) -> (202.2625, -106.5125) centre (201.7625, -106.5125) ccw
  line L268 (0, -80) -> (75, -80)
  line L269 (75, -80) -> (75, -100)
  line L270 (75, -100) -> (116.825, -100)
  line L271 (116.825, -100) -> (131.125, -114.3)
  line L272 (342.9, -100) -> (226.075, -100)
  line L273 (226.075, -100) -> (211.775, -114.3)
  line L274 (154.6375, -100.0125) -> (162.1375, -100.0125)
  line L275 (188.2625, -100.0125) -> (180.7625, -100.0125)
  line L276 (162.1375, 0) -> (162.1375, -114.3)
  line L277 (180.7625, -114.3) -> (180.7625, 0)
  line L278 (162.1375, 0) -> (0, 0)
  line L279 (0, 0) -> (0, -80)
  line L280 (131.125, -114.3) -> (162.1375, -114.3)
  line L281 (180.7625, -114.3) -> (211.775, -114.3)
  line L282 (342.9, -100) -> (342.9, 0)
  line L283 (342.9, 0) -> (180.7625, 0)
  line L284 (167.1375, 5) -> (-5, 5)
  line L285 (-5, 5) -> (-5, -85)
  line L286 (-5, -85) -> (70, -85)
  line L287 (70, -85) -> (70, -105)
  line L288 (70, -105) -> (114.7539, -105)
  line L289 (114.7539, -105) -> (129.0539, -119.3)
  line L290 (129.0539, -119.3) -> (167.1375, -119.3)
  line L291 (167.1375, 5) -> (167.1375, -119.3)
  line L292 (77, -98) -> (117.6534, -98)
  line L293 (117.6534, -98) -> (131.9534, -112.3)
  line L294 (131.9534, -112.3) -> (160.1375, -112.3)
  line L295 (160.1375, -2) -> (160.1375, -112.3)
  line L296 (160.1375, -2) -> (2, -2)
  line L297 (2, -2) -> (2, -78)
  line L298 (2, -78) -> (77, -78)
  line L299 (77, -78) -> (77, -98)
  line L300 (340.9, -2) -> (182.7625, -2)
  line L301 (182.7625, -112.3) -> (182.7625, -2)
  line L302 (182.7625, -112.3) -> (210.9466, -112.3)
  line L303 (225.2466, -98) -> (210.9466, -112.3)
  line L304 (340.9, -98) -> (225.2466, -98)
  line L305 (340.9, -98) -> (340.9, -2)
  line L306 (347.9, 5) -> (175.7625, 5)
  line L307 (175.7625, -119.3) -> (175.7625, 5)
  line L308 (175.7625, -119.3) -> (213.8461, -119.3)
  line L309 (228.1461, -105) -> (213.8461, -119.3)
  line L310 (347.9, -105) -> (228.1461, -105)
  line L311 (347.9, -105) -> (347.9, 5)
  dimension "d3" = 135
  dimension "d4" = 135
  dimension "d5" = 7.5
  dimension "d6" = 7.5
  dimension "d9" = -5
  dimension "d10" = -2
  dimension "d11" = 2
  dimension "d12" = -5
  constraint perpendicular L268 L269
  constraint perpendicular L233 L270
  constraint perpendicular L236 L272
  constraint midpoint L263 L274.start
  constraint perpendicular L263 L274
  constraint midpoint L266 L275.start
  constraint perpendicular L266 L275
  constraint perpendicular L276 L278
  constraint perpendicular L268 L279
  constraint perpendicular L276 L280
  constraint perpendicular L276 L281
  constraint perpendicular L257 L282
  constraint perpendicular L277 L283
  measures "d3" angle of L270 L271
  measures "d4" angle of L272 L273
  measures "d5" distance of L274.start L274.end
  measures "d6" distance of L275.start L275.end
extrude "Extrude1" add sketch "Sketch1" along normal blind 1.6 contours L268 L269 L270 L271 L276 L278 L279 L280 | L272 L273 L277 L281 L282 L283 | L292 L293 L294 L295 L296 L297 L298 L299 | L300 L301 L302 L303 L304 L305 makes body 1 at (149.1167, -49.0682, 0) makes body 2 at (193.7833, -49.0682, 0)
extrude "Extrude2" add sketch "Sketch1" against normal blind 15 separate body contours L268 L269 L270 L271 L276 L278 L279 L280 | L284 L285 L286 L287 L288 L289 L290 L291 makes body 3
extrude "Extrude3" add sketch "Sketch1" along normal blind 3 separate body contours L284 L285 L286 L287 L288 L289 L290 L291 makes body 4
combine "Combine1" operation add target body 3 tool bodies 4
extrude "Extrude4" add sketch "Sketch1" against normal blind 15 separate body contours L272 L273 L277 L281 L282 L283 | L306 L307 L308 L309 L310 L311 makes body 5
extrude "Extrude5" add sketch "Sketch1" along normal blind 3 separate body contours L306 L307 L308 L309 L310 L311 makes body 6
combine "Combine2" operation add target body 6 tool bodies 5
sketch "Sketch3" plane through (2, 0, 0) normal (1, 0, 0) x (0, 1, 0)
  line L0 (-2, 0) -> (-78, 0)
  line L1 (-78, 0) -> (-78, -15)
  line L2 (-78, -15) -> (-2, -15)
  line L3 (-2, -15) -> (-2, 0)
  line L4 (6, -13) -> (-120, -13)
  line L5 (-120, -13) -> (-120, -15)
  line L6 (-120, -15) -> (6, -15)
  line L7 (6, -15) -> (6, -13)
  constraint horizontal L4
  constraint vertical L5
  constraint horizontal L6
  constraint vertical L7
extrude "Extrude6" add sketch "Sketch3" along normal blind 160 contours L1 L2 L3 L4 L6 bodies 3
move_face "OffsetFaces1" offset 59 1 faces at (104.7125, -78, -13.6667) on bodies 3
extrude "Extrude7" cut 1 faces at (89.5846, -115.6667, -13) along direction (0, 0, -1) blind 9 on bodies 3 bodies 3
sketch "Sketch4" plane through (182.7625, 0, 0) normal (1, 0, 0) x (0, 1, 0)
  line L0 (-2, 0) -> (-112.3, 0)
  line L1 (-112.3, 0) -> (-112.3, -15)
  line L2 (-112.3, -15) -> (-2, -15)
  line L3 (-2, -15) -> (-2, 0)
  line L4 (-120, -15) -> (8, -15)
  line L5 (8, -15) -> (8, -13)
  line L6 (8, -13) -> (-120, -13)
  line L7 (-120, -13) -> (-120, -15)
  constraint horizontal L4
  constraint vertical L5
  constraint horizontal L6
  constraint vertical L7
extrude "Extrude8" add sketch "Sketch4" along normal blind 170 contours L1 L2 L3 L4 L6 bodies 6
extrude "Extrude9" cut 1 faces at (267.2515, -109.8667, -13) along direction (0, 0, -1) blind 15 on bodies 6 bodies 6
sketch "Sketch5" plane through (0, 5, 0) normal (0, 1, 0) x (-1, 0, 0)
  line L0 (-167.1375, 3) -> (-167.1375, -15)
  line L1 (-167.1375, -15) -> (5, -15)
  line L2 (5, -15) -> (5, 3)
  line L3 (5, 3) -> (-167.1375, 3)
  circle A0 centre (-200, -5) radius 4
  circle A1 centre (-185, -5) radius 4
  circle A2 centre (-157, -5) radius 4
extrude "Extrude10" cut sketch "Sketch5" against normal blind 6 contours A0 | A1 | A2 bodies 3 6
extrude "Extrude11" cut 2 faces at (185.0996, -1, -7.1156) (200.0996, -1, -7.1156) along direction (0, -1, 0) blind 1 on bodies 6 bodies 6
extrude "Extrude12" cut 1 faces at (157.0996, -1, -7.1156) along direction (0, -1, 0) blind 1 on bodies 3 bodies 3
extrude "Extrude13" cut 2 faces at (77.3792, -25, -15) (250.6029, -31.6667, -15) along direction (0, 0, 1) blind 2 on bodies 3 6 bodies 3 6
extrude "Extrude14" add 2 faces at (235.475, 2.6667, -13) (54.7125, 2.6667, -13) along direction (0, 0, -1) blind 10 on bodies 3 6 bodies 6 3
sketch "Sketch6" plane through (2, 0, 0) normal (1, 0, 0) x (0, 1, 0)
  line L0 (-2, -23) -> (-2, 0)
  line L1 (-2, 0) -> (-78, 0)
  line L2 (-78, 0) -> (-78, -23)
  line L3 (-78, -23) -> (-2, -23)
  line L4 (-105, -25) -> (10, -25)
  line L5 (10, -25) -> (10, -21)
  line L6 (10, -21) -> (-105, -21)
  line L7 (-105, -21) -> (-105, -25)
  constraint horizontal L4
  constraint vertical L5
  constraint horizontal L6
  constraint vertical L7
extrude "Extrude15" add sketch "Sketch6" along normal blind 159 contours L0 L2 L3 L6 bodies 3
move_face "OffsetFaces2" offset 41 1 faces at (104.7125, -78, -21.6667) on bodies 3
extrude "Extrude16" cut 1 faces at (106.836, -114.3333, -21) along direction (0, 0, -1) blind 11 on bodies 3 bodies 3
delete_face "DeleteFace1" 1 faces at (199.3054, 2.6667, -1.0608) on bodies 6
delete_face "DeleteFace2" 1 faces at (188.9888, 2.6667, -5.2987) on bodies 6
sketch "Sketch7" plane through (182.7625, 0, 0) normal (1, 0, 0) x (0, 1, 0)
  line L0 (-2, -23) -> (-2, 0)
  line L1 (-2, 0) -> (-112.3, 0)
  line L2 (-112.3, 0) -> (-112.3, -23)
  line L3 (-112.3, -23) -> (-2, -23)
  line L4 (-125, -25) -> (11, -25)
  line L5 (11, -25) -> (11, -21)
  line L6 (11, -21) -> (-125, -21)
  line L7 (-125, -21) -> (-125, -25)
  constraint horizontal L4
  constraint vertical L5
  constraint horizontal L6
  constraint vertical L7
extrude "Extrude17" add sketch "Sketch7" along normal blind 160 contours L0 L2 L3 L6 bodies 6
extrude "Extrude18" cut 1 faces at (263.9182, -109.8667, -21) along direction (0, 0, -1) blind 5 on bodies 6 bodies 6
delete_face "DeleteFace3" 1 faces at (160.9889, 2.6667, -5.2983) on bodies 3
sketch "Sketch8" plane through (0, 5, 0) normal (0, 1, 0) x (-1, 0, 0)
  line L0 (5, -23) -> (5, 3)
  line L1 (5, 3) -> (-167.1375, 3)
  line L2 (-167.1375, 3) -> (-167.1375, -23)
  line L3 (-167.1375, -23) -> (5, -23)
  line L4 (-167.1375, 3) -> (-154.1375, -10)
  line L5 (-167.1375, 3) -> (-148.7527, 3) construction
  line L6 (-175.7625, 3) -> (-188.7625, -10)
  line L7 (-175.7625, 3) -> (-157.3777, 3) construction
  circle A0 centre (-188.7625, -10) radius 7.5
  circle A1 centre (-154.1375, -10) radius 7.5
  dimension "d49" = 45
  dimension "d50" = 135
  dimension "d51" = 15
  dimension "d52" = 15
  constraint horizontal L5
  constraint coincident L1.end L2.start
  constraint horizontal L7
  constraint coincident L6.end A0.centre
  constraint coincident L4.end A1.centre
  measures "d49" angle of L4 L5
  measures "d50" angle of L6 L7
  measures "d51" diameter of A0
  measures "d52" diameter of A1
extrude "Extrude19" cut sketch "Sketch8" against normal blind 17 contours A0 | A1 bodies 3 6
extrude "Extrude20" add 2 faces at (249.6364, -34, -23) (235.475, 2.6667, -23) along direction (0, 0, -1) blind 4 on bodies 6 bodies 6
extrude "Extrude21" cut 1 faces at (249.6364, -34, -21) along direction (0, 0, -1) blind 2 on bodies 6 bodies 6
extrude "Extrude22" cut 1 faces at (249.6364, -34, -23) along direction (0, 0, -1) blind 2 on bodies 6 bodies 6
extrude "Extrude23" add 1 faces at (77.3792, -25, -23) along direction (0, 0, -1) blind 4 on bodies 3 bodies 3
extrude "Extrude24" cut 1 faces at (79.7125, -27.3333, -21) along direction (0, 0, -1) blind 4 on bodies 3 bodies 3
combine "Combine3" operation add target body 6 tool bodies 3 makes body 7 at (77.3792, -25, -27)
extrude "Extrude25" add 1 faces at (182.5865, -12, -11.2309) along direction (0, 1, 0) blind 17 on bodies 6 bodies 6
extrude "Extrude26" add 1 faces at (160.3309, -12, -8.8003) along direction (0, 1, 0) blind 17 on bodies 7 bodies 7
